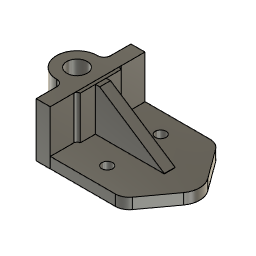
A3 (Autodesk Fusion 360 design; units mm, degrees)
Autodesk Fusion 360 part; units mm, degrees
note: some values were not read from the file. Set by a fixed rule: which sketch regions a step uses.
sketch "Sketch3" plane through (0, 0, 0) normal (0, 0, 1) x (1, 0, 0)
  line L0 (33.5, -44) -> (-33.5, -44)
  line L1 (-33.5, -44) -> (-33.5, 44)
  line L2 (-33.5, 44) -> (33.5, 44)
  line L3 (33.5, -44) -> (-33.5, 44) construction
  line L4 (-33.5, -44) -> (33.5, 44) construction
  circle A0 centre (0, 25) radius 5
  circle A1 centre (0.3763, -25) radius 5
  line L5 (33.5, -44) -> (57.4793, -11.2043)
  line L6 (57.476, 11.2288) -> (33.5, 44)
  arc A2 (57.4793, -11.2043) -> (57.476, 11.2288) centre (42.1418, 0.01) ccw
  line L7 (33.5, 44) -> (33.5, -44)
  dimension "d5" = 67
  dimension "d6" = 88
  dimension "d7" = 10
  dimension "d8" = 10
  dimension "d9" = 50
  dimension "d10" = 19
  dimension "d55" = 19
  constraint horizontal L0
  constraint perpendicular L0 L1
  constraint parallel L0 L2
  constraint coincident L3 origin
  constraint coincident L4 origin
  constraint tangent L5 A2
  constraint tangent L6 A2
  constraint perpendicular L0 L7
  measures "d5" distance of L1.end L2.end
  measures "d6" distance of L0.end L1.end
  measures "d7" diameter of A0
  measures "d8" diameter of A1
  measures "d9" vertical distance of A0.centre A1.centre
  measures "d10" distance of L2 A0.centre
  measures "d55" radius of A2
extrude "Extrude1" add sketch "Sketch3" along normal blind 10 contours L0 L1 L2 L7 makes body 1
sketch "Sketch4" plane through (0, 0, 0) normal (0, 0, 1) x (1, 0, 0)
  line L0 (-33.5117, 43.8664) -> (-46.5117, 43.8664)
  line L1 (-46.5117, -44.1336) -> (-33.5117, -44.1336)
  line L2 (-33.5117, -44.1336) -> (-33.5117, 43.8664)
  line L3 (-46.5117, 43.8664) -> (-46.5117, 24.9992)
  line L4 (-46.5117, -24.9992) -> (-46.5117, -44.1336)
  arc A0 (-52.5605, 18.9994) -> (-52.5605, -18.9994) centre (-52.715, 0) ccw
  circle A1 centre (-52.715, 0) radius 9.5
  arc A2 (-52.5605, 18.9994) -> (-46.5117, 24.9992) centre (-52.5117, 24.9992) ccw
  arc A3 (-46.5117, -24.9992) -> (-52.5605, -18.9994) centre (-52.5117, -24.9992) ccw
  dimension "d16" = 19
  dimension "d17" = 19
  dimension "d18" = 6
  dimension "d19" = 6
  constraint horizontal L0
  constraint vertical L3
  constraint horizontal L1
  constraint vertical L2
  constraint collinear L3 L4
  constraint concentric A0 A1
  constraint tangent L3 A2
  constraint tangent A0 A2
  constraint tangent L4 A3
  constraint tangent A0 A3
  measures "d16" radius of A0
  measures "d17" diameter of A1
  measures "d18" radius of A2
  measures "d19" radius of A3
extrude "Extrude2" add sketch "Sketch4" along normal blind 50 separate body makes body 2
sketch "Sketch5" plane through (-33.5117, 0, 0) normal (1, 0, 0) x (0, 1, 0)
  line L0 (-44.1336, 0) -> (43.8664, 0)
  line L1 (43.8664, 0) -> (43.8664, 50)
  line L2 (43.8664, 50) -> (-44.1336, 50)
  line L3 (-44.1336, 50) -> (-44.1336, 0)
  line L4 (-19.1336, 49.9963) -> (18.8664, 49.9963)
  line L5 (18.8664, 49.9963) -> (18.8664, 9.9944)
  line L6 (18.8664, 9.9944) -> (-19.1336, 9.9944)
  line L7 (-19.1336, 9.9944) -> (-19.1336, 49.9963)
  dimension "d22" = 38
  dimension "d23" = 25
  constraint horizontal L4
  constraint vertical L5
  constraint horizontal L6
  constraint vertical L7
  measures "d22" distance of L4.start L4.end
  measures "d23" distance of L3 L7
extrude "Extrude4" add sketch "Sketch5" along normal blind 3 contours L4 L5 L6 L7 bodies 2
fillet "Fillet2" radius 3 1 edges at (-33.5117, -19.1336, 29.9954) on bodies 2
fillet "Fillet3" radius 3 1 edges at (-33.5117, 18.8664, 29.9954) on bodies 2
extrude "Extrude3" cut sketch "Sketch5" along normal blind 3 contours L4 L5 L6 L7 bodies 1
sketch "Sketch8" plane through (0, 0, 10) normal (0, 0, 1) x (-1, 0, 0)
  line L0 (30.5117, 19.1336) -> (33.5, 19.1336)
  line L1 (33.5, 19.1336) -> (33.5, 44)
  line L2 (33.5, 44) -> (-33.5, 44)
  line L3 (-33.5, -44) -> (33.5, -44)
  line L4 (33.5, -44) -> (33.5, -18.8664)
  line L5 (33.5, -18.8664) -> (30.5117, -18.8664)
  line L6 (30.5117, -18.8664) -> (30.5117, 19.1336)
  circle A0 centre (-0.3763, 25) radius 5
  circle A1 centre (0, -25) radius 5
  line L7 (30.5117, -4.8664) -> (-33.5, -4.8664)
  line L8 (-33.5, -4.8664) -> (-33.5, 5.1336)
  line L9 (-33.5, 5.1336) -> (30.5117, 5.1336)
  line L10 (30.5117, 5.1336) -> (30.5117, -4.8664)
  line L11 (-33.5, 44) -> (-33.5, -44)
  dimension "d38" = 14
  dimension "d39" = 10
  constraint horizontal L7
  constraint vertical L8
  constraint horizontal L9
  constraint vertical L10
  measures "d38" vertical distance of L0.start L8.end
  measures "d39" distance of L7.end L8.end
extrude "Extrude5" add sketch "Sketch8" along normal blind 40 contours L6 L7 L8 L9 L10 L11 bodies 1 2
chamfer "Chamfer1" distance 60 angle 33.5 1 edges at (33.5, -0.1336, 50) measured on face at (12.1628, -1.8003, 50) on bodies 1
extrude "Extrude7" add sketch "Sketch3" along normal blind 10 contours L5 L6 A2 L7 bodies 1
fillet "Fillet8" radius 13 1 edges at (33.5, -44, 5) on bodies 1
fillet "Fillet9" radius 13 1 edges at (33.5, 44, 5) on bodies 1
equation "d10 = ( ( 88 - 50 ) / 2 ) * 1 mm"
